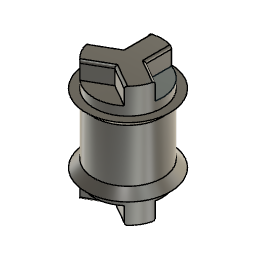
q5_fusion _final (Autodesk Fusion 360 design; units mm, degrees)
Autodesk Fusion 360 part; units mm, degrees
note: some values were not read from the file. Chosen so that the rebuilt part matches the saved one: the sign of a taper; which pieces of a blend or face edit are solid. Set by a fixed rule: which sketch regions a step uses.
sketch "Sketch1" plane through (0, 0, 0) normal (0, 0, 1) x (1, 0, 0)
  circle A0 centre (0, 0) radius 15
  dimension "d1" = 30
  constraint coincident A0.centre origin
  measures "d1" diameter of A0
extrude "Extrude1" add sketch "Sketch1" along normal blind 11 makes body 1
sketch "Sketch2" plane through (0, 0, 11) normal (0, 0, 1) x (-1, 0, 0)
  circle A0 centre (0, 0) radius 15
  circle A1 centre (0, 0) radius 18.5
  dimension "d4" = 37
  constraint concentric A0 A1
  measures "d4" diameter of A1
extrude "Extrude2" add sketch "Sketch2" along normal blind 4.1 separate body makes body 2
sketch "Sketch3" plane through (0, 0, 11) normal (0, 0, 1) x (-1, 0, 0)
  circle A0 centre (0, 0) radius 15
draft "Draft1" angle -45 neutral plane through (0, 0, 15.1) pull (0, 0, 1) 1 faces at (-18.477, 0.9221, 13.7333) on bodies 2
extrude "Extrude3" add sketch "Sketch3" along normal blind 8 bodies 1 2
sketch "Sketch4" plane through (0, 0, 19) normal (0, 0, 1) x (-1, 0, 0)
  circle A0 centre (0, 0) radius 15
  line L0 (5, 0) -> (5, -14.1421)
  line L1 (-5, -14.1421) -> (-5, 0)
  line L2 (5, 0) -> (-5, 0)
  constraint parallel L0 L1
  constraint coincident A0.centre origin
  constraint coincident A0 L1.start
  constraint coincident A0 L0.end
extrude "Extrude4" add sketch "Sketch4" along normal blind 7.5 contours A0 L0 L1 L2 picked at (0.3396, -4.9885) bodies 1
pattern_circular "C-Pattern1" count 3 over 360 about axis through (0, 0, 15.1) along (0, 0, 1) of "Extrude4"
sketch "Sketch5" plane through (0, 0, 19) normal (0, 0, 1) x (-1, 0, 0)
  line L0 (-5, -2.8868) -> (-14.7474, 2.7409)
  arc A0 (-14.7474, 2.7409) -> (-5, -14.1421) centre (0, 0) ccw
  line L1 (-5, -14.1421) -> (-5, -2.8868)
fillet "Fillet1" radius 1 6 edges at (4.8737, -8.5873, 26.5) (-4.8737, -8.5873, 26.5) (-9.8737, 0.0729, 26.5) (-5, 8.5144, 26.5) (5, 8.5144, 26.5) (9.8737, 0.0729, 26.5) on bodies 1
extrude "Extrude5" add 1 faces at (3.6653, 3.4009, 0) along direction (0, 0, -1) blind 11 on bodies 1 bodies 1
sketch "Sketch6" plane through (0, 0, -11) normal (0, 0, -1) x (1, 0, 0)
  circle A0 centre (0, 0) radius 15
sketch "Sketch7" plane through (0, 0, -11) normal (0, 0, -1) x (1, 0, 0)
sketch "Sketch8" plane through (0, 0, -11) normal (0, 0, -1) x (1, 0, 0)
  circle A0 centre (0, 0) radius 18.5
  dimension "d20" = 37
  constraint coincident A0.centre origin
  measures "d20" diameter of A0
sketch "Sketch14" plane through (0, 0, -11) normal (0, 0, -1) x (1, 0, 0)
  circle A0 centre (0, 0) radius 15
  circle A1 centre (0, 0) radius 18.5
  dimension "d36" = 37
  constraint coincident A0.centre A1.centre
  measures "d36" diameter of A1
extrude "Extrude9" add sketch "Sketch14" along normal blind 4.1 separate body makes body 3
draft "Draft3" angle -45 neutral plane through (0, 0, -15.1) pull (0, 0, -1) 1 faces at (18.4081, 1.842, -12.3667) on bodies 3
extrude "Extrude10" add 1 faces at (3.6653, 3.4009, -11) along direction (0, 0, -1) blind 8 on bodies 1 bodies 1 3
sketch "Sketch15" plane through (0, 0, 0) normal (0, 1, 0) x (1, 0, 0)
sketch "Sketch16" plane through (0, 0, -19) normal (0, 0, -1) x (1, 0, 0)
  circle A0 centre (0, 0) radius 15
  line L0 (5, -14.1421) -> (5, 0)
  line L1 (-5, 0) -> (-5, -14.1421)
  line L2 (5, 0) -> (-5, 0) construction
  line L3 (5, 0) -> (-5, 0)
  constraint parallel L0 L1
  constraint coincident A0.centre origin
  constraint coincident A0 L0.start
  constraint coincident A0 L1.end
extrude "Extrude11" add sketch "Sketch16" along normal blind 7.5 contours A0 L0 L1 L3 picked at (0.3396, -4.9885) bodies 1
pattern_circular "C-Pattern3" count 3 over 360 about axis through (0, 0, -15.1) along (0, 0, -1) of "Extrude11"
fillet "Fillet3" radius 1 6 edges at (-9.8737, 0.0729, -26.5) (-4.8737, -8.5873, -26.5) (4.8737, -8.5873, -26.5) (9.8737, 0.0729, -26.5) (5, 8.5144, -26.5) (-5, 8.5144, -26.5) on bodies 1
